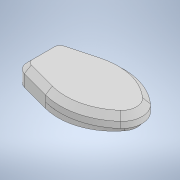
# Autodesk Inventor part: FS-00-SLBV8
Saved by Autodesk Inventor 2022.2 (Build 262287000, 287)
## iProperties
Created: 2021-12-12
Part Number: FS-00-SLBV8
Material: Generic
Document SubType Name: Modeling
Designer: Frank
Density: 1 g/cm^3
Appearance: Default
Author: Frank
Autodesk Inventor part; units mm, degrees
ref_plane "YZ Plane" through (0, 0, 0) normal (1, 0, 0) x (0, 1, 0)
ref_plane "XZ Plane" through (0, 0, 0) normal (0, 1, 0) x (-1, 0, 0)
ref_plane "XY Plane" through (0, 0, 0) normal (0, 0, 1) x (1, 0, 0)
sketch "Sketch1" plane through (0, 0, 0) normal (0, 1, 0) x (-1, 0, 0)
  circle A0 centre (0, 0) radius 5.5
  line L0 (0, 0) -> (30, 0) construction
  line L1 (30, -7) -> (30, 7)
  line L2 (30, -7) -> (16.7292, -10.5559)
  arc A1 (-4.3821, -3.3237) -> (16.7292, -10.5559) centre (11.5528, 8.7626) ccw
  line L3 (30, 7) -> (16.7292, 10.5559)
  arc A2 (16.7292, 10.5559) -> (-4.3821, 3.3237) centre (11.5528, -8.7626) ccw
  circle A3 centre (0, 0) radius 7.25
  arc A4 (16.7292, 10.5559) -> (-4.8424, 5.3957) centre (10.7046, -11.928) ccw
  arc A5 (-4.8424, -5.3957) -> (16.7292, -10.5559) centre (10.7046, 11.928) ccw
  point P0 (1.7838, 5.2027)
  point P1 (1.7838, -5.2027)
  point P2 (16.7292, 10.5559)
  point P3 (30, 9.4853)
  point P4 (30, -9.4853)
  point P5 (30, -9.4752)
  point P6 (30, 9.4752)
  dimension "d0" = 11
  dimension "d1" = 30
  dimension "d2" = 14
  dimension "d5" = 30
  dimension "d10" = 14.5
  dimension "d52" = 20
  constraints: 15 point on circle, 8 end point, 7 tangent, 6 centre point, 2 coincident, 1 equal radius, 1 horizontal, 1 midpoint, 1 symmetric about line, 1 vertical, 1 other
  measures "d0" diameter of A0
  measures "d1" distance of L0.start L0.end
  measures "d2" distance of L1.start L1.end
  measures "d5" angle of L3 L2
  measures "d10" diameter of A3
  measures "d52" radius of A2
extrude "Extrusion1" add sketch "Sketch1" against normal blind 2 contours A0 | A0 A2 A3 A1 | A2 L3 L1 L2 A1 A3 picked at (6.6012, -0.5586)
extrude "Extrusion2" add sketch "Sketch1" along normal blind 4.2
fillet "Fillet1" radius 4 2 edges at (-30, 1.1, 7) (-30, 1.1, -7)
chamfer "Chamfer1" distance 2 angle 45 8 edges at (-30, 4.2, 0) (-29.1734, 4.2, 6.3657) (-21.8822, 4.2, 9.1752) (-5.2893, 4.2, 10.7104) (7.25, 4.2, 0) (-5.2893, 4.2, -10.7104) (-21.8822, 4.2, -9.1752) (-29.1734, 4.2, -6.3657)
sketch "Sketch9" plane through (0, -2, 0) normal (0, -1, 0) x (1, 0, 0)
  arc A0 (-27.0353, 7.7944) -> (-30, 3.9307) centre (-26, 3.9307) ccw projected
  line L0 (-30, 3.9307) -> (-30, -3.9307) projected
  arc A1 (-30, -3.9307) -> (-27.0353, -7.7944) centre (-26, -3.9307) ccw projected
  arc A2 (6.1782, -6.8842) -> (6.1782, 6.8842) centre (0, 0) ccw projected
  line L1 (-32, -3.9307) -> (-32, 3.9307) projected
  line L2 (-27.5363, -9.7307) -> (-33.6527, -8.0918)
  arc A3 (-36.9536, -3.79) -> (-33.6527, -8.0918) centre (-32.5, -3.79) ccw
  line L3 (-36.9536, -3.79) -> (-36.9536, 4.2596)
  arc A4 (-33.0372, 8.6806) -> (-36.9536, 4.2596) centre (-32.5, 4.2596) ccw
  line L4 (-32, 3.9307) -> (-32, -3.9307) projected
  line L5 (-26.7661, 9.4426) -> (-33.0372, 8.6806)
  arc A5 (-17.2468, -12.4878) -> (6.1782, -6.8842) centre (-10.7046, 11.928) ccw projected
  line L6 (-26.5589, -7.4525) -> (-33.0176, -5.7218)
  arc A6 (-34.5, -3.79) -> (-33.0176, -5.7218) centre (-32.5, -3.79) ccw
  line L7 (-34.5, -3.79) -> (-34.5, 4.2596)
  arc A7 (-33.0176, 6.1914) -> (-34.5, 4.2596) centre (-32.5, 4.2596) ccw
  line L8 (-33.0176, 6.1914) -> (-27.0353, 7.7944)
  arc A8 (4.3821, 3.3237) -> (-16.7292, 10.5559) centre (-11.5528, -8.7626) ccw projected
  arc A9 (-16.7292, -10.5559) -> (4.3821, -3.3237) centre (-11.5528, 8.7626) ccw projected
  arc A10 (4.3821, -3.3237) -> (4.3821, 3.3237) centre (0, 0) ccw projected
  arc A11 (4.3821, 3.3237) -> (-16.7292, 10.5559) centre (-11.5528, -8.7626) ccw projected
  line L9 (-16.7292, 10.5559) -> (-27.0353, 7.7944) projected
  line L10 (-27.0353, -7.7944) -> (-16.7292, -10.5559) projected
  arc A12 (-17.2468, -12.4878) -> (6.1782, -6.8842) centre (-10.7046, 11.928) ccw projected
  line L11 (-17.2468, -12.4878) -> (-27.5529, -9.7262) projected
  arc A13 (-32, -3.9307) -> (-27.5529, -9.7262) centre (-26, -3.9307) ccw projected
  arc A14 (-27.5529, 9.7262) -> (-32, 3.9307) centre (-26, 3.9307) ccw projected
  line L12 (-27.5529, 9.7262) -> (-17.2468, 12.4878) projected
  arc A15 (6.1782, 6.8842) -> (-17.2468, 12.4878) centre (-10.7046, -11.928) ccw projected
  line L13 (-27.5529, -9.7262) -> (-17.2468, -12.4878) projected
  line L14 (-27.0353, 7.7944) -> (-16.7292, 10.5559) projected
  point P0 (-27.5529, -9.7262)
  point P1 (-31.5927, -6.1037)
  point P2 (-31.355, 6.6369)
  point P3 (-28.9, 9.1833)
  dimension "d90" = 2.5
  dimension "d91" = 2
  constraints: 12 end point, 8 point on circle, 8 tangent, 4 centre point, 2 coincident, 2 collinear, 2 parallel, 1 equal radius, 1 vertical
  measures "d90" distance between parallel lines of L7 L1
  measures "d91" radius of A6
sketch "Sketch11" plane through (0, 6.1, 0) normal (0, 1, 0) x (1, 0, 0)
  arc A0 (4.0599, -4.5238) -> (4.0599, 4.5238) centre (0, 0) ccw projected
  line L0 (-28.8284, -3.9307) -> (-28.8284, 3.9307) projected
  line L1 (-26.7321, 6.6627) -> (-16.4259, 9.4243) projected
  arc A1 (4.0599, 4.5238) -> (-16.4259, 9.4243) centre (-10.7046, -11.928) ccw projected
  arc A2 (-16.4259, -9.4243) -> (4.0599, -4.5238) centre (-10.7046, 11.928) ccw projected
  line L2 (-16.4259, -9.4243) -> (-26.7321, -6.6627) projected
  arc A3 (-28.8284, -3.9307) -> (-26.7321, -6.6627) centre (-26, -3.9307) ccw projected
  arc A4 (-26.7321, 6.6627) -> (-28.8284, 3.9307) centre (-26, 3.9307) ccw projected
  dimension "d75" = 1
  dimension "d76" = 1
  dimension "d77" = 1
  dimension "d78" = 10
  dimension "d79" = 80
  constraints: 18 end point, 15 point on circle, 4 centre point, 4 coincident, 4 parallel, 4 tangent, 3 midpoint, 1 equal radius, 1 horizontal, 1 horizontal alignment, 1 perpendicular, 1 point on line, 1 other
  measures "d75" distance from line of L1 point (-11.375, -0.5)
  measures "d76" radial gap between concentric circles of A1 A2
  measures "d77" radial gap between concentric circles of A3 A4
  measures "d78" distance of point (0, 0) A3.centre
sketch "Sketch16" plane through (0, 11.1, 0) normal (0, 1, 0) x (1, 0, 0)
  point P0 (0, 0)
sketch "Sketch15" plane through (-28, 4.1, -3.9307) normal (0, -1, 0) x (1, 0, 0)
  point P0 (28, 3.9307)
  point P1 (28, 3.9307)
body "Solid1"
